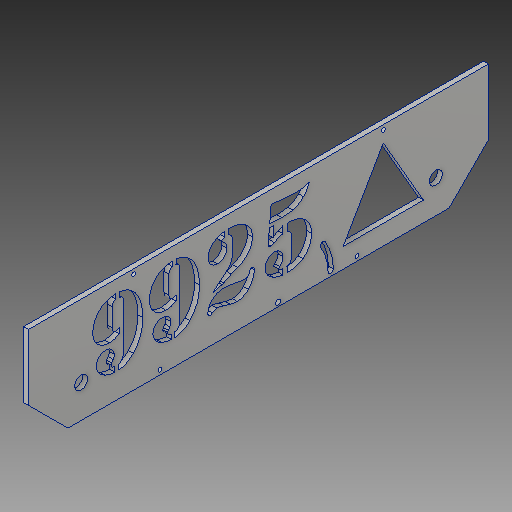
# Autodesk Inventor part: DriveTrain3.0
Saved by Autodesk Inventor 2019 (Build 230136000, 136)
## iProperties
Created: 2017-07-22
Part Number: DriveTrain3.0
Material: Aluminum 6061
Document SubType Name: Modeling
Designer: User
Density: 2.7 g/cm^3
Appearance: Aluminum - Flat
Mass: 590.045 g
Surface Area: 982.684 cm^2
Volume: 218.535 cm^3
Author: User
Autodesk Inventor part; units mm, degrees
ref_plane "YZ Plane" through (0, 0, 0) normal (1, 0, 0) x (0, 1, 0)
ref_plane "XZ Plane" through (0, 0, 0) normal (0, 1, 0) x (-1, 0, 0)
ref_plane "XY Plane" through (0, 0, 0) normal (0, 0, 1) x (1, 0, 0)
sketch "Sketch1" plane through (0, 0, 0) normal (1, 0, 0) x (0, 1, 0)
  line L0 (0, 0) -> (101.6, 0)
  line L1 (101.6, 0) -> (101.6, -444.5)
  line L2 (101.6, -444.5) -> (0, -444.5)
  line L3 (0, -444.5) -> (0, 0)
  circle A0 centre (31.75, -50.8) radius 6.3627
  circle A1 centre (31.75, -393.7) radius 6.3627
  circle A2 centre (86.2838, -165.5318) radius 1.5875
  circle A3 centre (70.2818, -165.5318) radius 1.5875
  circle A4 centre (15.3162, -278.9682) radius 1.5875
  circle A5 centre (31.3182, -278.9682) radius 1.5875
  dimension "d0" = 101.6
  dimension "d1" = 444.5
  dimension "d2" = 12.7254
  dimension "d3" = 31.75
  dimension "d4" = 50.8
  dimension "d5" = 50.8
  dimension "d22" = 165.5318
  dimension "d23" = 3.175
  dimension "d24" = 15.3162
  dimension "d25" = 3.175
  dimension "d26" = 16.002
  dimension "d27" = 165.5318
  dimension "d28" = 3.175
  dimension "d29" = 15.3162
  dimension "d30" = 165.5318
  dimension "d31" = 3.175
  dimension "d32" = 16.002
  dimension "d33" = 165.5318
  constraints: 8 end point, 6 centre point, 2 parallel, 1 horizontal, 1 perpendicular
  measures "d0" distance of L1.end L2.end
  measures "d1" distance of L0.end L1.end
  measures "d2" diameter of A0
  measures "d3" distance from line of L3 A0.centre
  measures "d4" distance from line of L0 A0.centre
  measures "d5" distance from line of L2 A1.centre
  measures "d22" distance from line of L0 A2.centre
  measures "d23" diameter of A2
  measures "d24" distance from line of L1 A2.centre
  measures "d25" diameter of A3
  measures "d26" distance of A2.centre A3.centre
  measures "d27" distance from line of L0 A3.centre
  measures "d28" diameter of A4
  measures "d29" distance from line of L3 A4.centre
  measures "d30" distance from line of L2 A4.centre
  measures "d31" diameter of A5
  measures "d32" distance of A5.centre A4.centre
  measures "d33" distance from line of L2 A5.centre
extrude "Extrusion1" add sketch "Sketch1" along normal blind 4.7625 contours L0 L1 L2 L3 | A2 | A3 | A4 | A5
chamfer "Chamfer1" distance 38.1 angle 45 1 edges at (2.3813, 0, 0)
chamfer "Chamfer2" distance 38.1 angle 45 1 edges at (2.3813, 0, -444.5)
sketch "Sketch8" plane through (4.7625, 0, 0) normal (1, 0, 0) x (0, 0, -1)
  line L0 (444.5, 38.1) -> (406.4, 0) projected
  line L1 (444.5, 38.1) -> (444.5, 101.6) projected
  line L2 (444.5, 101.6) -> (0, 101.6) projected
  line L3 (0, 101.6) -> (0, 38.1) projected
  line L4 (38.1, 0) -> (0, 38.1) projected
  line L5 (38.1, 0) -> (406.4, 0) projected
  circle A0 centre (393.7, 31.75) radius 6.3627 projected
  circle A1 centre (50.8, 31.75) radius 6.3627 projected
  point P0 (0, 0)
  point P1 (101.6, 97.155)
  point P2 (342.9, 97.155)
  point P3 (127, 4.445)
  point P4 (317.5, 4.445)
  dimension "d110" = 4.445
  dimension "d111" = 4.445
  dimension "d112" = 101.6
  dimension "d113" = 101.6
  dimension "d114" = 4.445
  dimension "d115" = 4.445
  dimension "d123" = 127
  dimension "d124" = 127
  measures "d110" distance from line of L2 point (342.9, 97.155)
  measures "d111" distance from line of L2 point (101.6, 97.155)
  measures "d112" distance from line of L3 point (101.6, 97.155)
  measures "d113" distance from line of L1 point (342.9, 97.155)
  measures "d114" distance from line of L5 point (317.5, 4.445)
  measures "d115" distance from line of L5 point (127, 4.445)
  measures "d123" distance from line of L1 point (317.5, 4.445)
  measures "d124" distance from line of L3 point (127, 4.445)
hole "Hole3" at (4.7625, 97.155, -101.6) at (4.7625, 97.155, -342.9) at (4.7625, 4.445, -127) at (4.7625, 4.445, -317.5) direction (-1, 0, 0) diameter 3.81 depth 25.4 tip angle 118
sketch "Sketch9" plane through (4.7625, 0, 0) normal (1, 0, 0) x (0, 0, -1)
  line L0 (444.5, 38.1) -> (444.5, 101.6) projected
  line L1 (38.1, 0) -> (406.4, 0) projected
  arc A0 (292.0841, 5.08) -> (284.536, 30.48) centre (241.3, 3.81) ccw construction
  arc A1 (294.6233, 5.1435) -> (286.6978, 31.8135) centre (241.3, 3.81) ccw
  arc A2 (289.5449, 5.0165) -> (282.3742, 29.1465) centre (241.3, 3.81) ccw
  arc A3 (289.5449, 5.0165) -> (294.6233, 5.1435) centre (292.0841, 5.08) ccw
  arc A4 (286.6978, 31.8135) -> (282.3742, 29.1465) centre (284.536, 30.48) ccw
  point P0 (0, 0)
  dimension "d125" = 203.2
  dimension "d126" = 3.81
  dimension "d134" = 50.8
  dimension "d135" = 5.08
  dimension "d139" = 5.08
  dimension "d140" = 25.4
  constraints: 10 point on circle, 5 centre point, 4 tangent, 1 coincident
  measures "d125" distance from line of L0 point (241.3, 3.81)
  measures "d126" distance from line of point (241.3, 3.81) L1
  measures "d134" radius of A0
  measures "d135" diameter of A4
  measures "d139" distance from line of L1 A0.start
  measures "d140" vertical distance of A0.start A0.end
hole "Hole4" at (4.7625, 3.81, -241.3) direction (-1, 0, 0) diameter 5.08 end through all
extrude "Extrusion6" cut sketch "Sketch9" against normal through all
sketch "Sketch10" plane through (4.7625, 0, 0) normal (1, 0, 0) x (0, 0, -1)
  line L0 (59.5129, 89.2474) -> (313.2288, 89.2474) construction
  line L1 (313.2288, 89.2474) -> (313.2288, 0) construction
  line L2 (313.2288, 0) -> (59.5129, 0) construction
  line L3 (59.5129, 0) -> (59.5129, 89.2474) construction
  line L4 (86.7981, 24.204) -> (86.7981, 28.8893)
  spline S0 degree 2 poles (86.7981, 28.8893) (88.2863, 29.3303) (89.8297, 30.3776) (90.381, 31.3698) knots 0 0 0 1 2 2 2
  spline S1 degree 2 poles (90.381, 31.3698) (91.5385, 33.299) (91.5385, 35.6141) knots 0 0 0 1 1 1
  line L5 (91.5385, 35.6141) -> (91.5385, 78.5538)
  spline S2 degree 2 poles (91.5385, 78.5538) (91.5385, 80.7036) (91.2629, 82.5226) (90.7668, 83.184) knots 0 0 0 1 2 2 2
  spline S3 degree 2 poles (90.7668, 83.184) (89.9951, 84.1211) (87.9005, 84.7274) knots 0 0 0 1 1 1
  line L6 (87.9005, 84.7274) -> (87.9005, 89.2474)
  spline S4 degree 2 poles (87.9005, 89.2474) (92.3653, 88.8064) (100.1926, 84.4518) (103.2243, 80.7587) knots 0 0 0 1 2 2 2
  spline S5 degree 2 poles (103.2243, 80.7587) (106.6969, 76.6797) (110.4452, 63.8364) (110.4452, 56.3398) knots 0 0 0 1 2 2 2
  spline S6 degree 2 poles (110.4452, 56.3398) (110.4452, 40.3546) (101.295, 31.0391) knots 0 0 0 1 1 1
  spline S7 degree 2 poles (101.295, 31.0391) (98.0429, 27.7869) (90.4912, 24.204) (86.7981, 24.204) knots 0 0 0 1 2 2 2
  line L7 (87.9005, 59.3715) -> (87.9005, 54.0247)
  spline S8 degree 2 poles (87.9005, 54.0247) (82.8293, 51.2687) (78.0889, 51.2687) knots 0 0 0 1 1 1
  spline S9 degree 2 poles (78.0889, 51.2687) (75.1674, 51.2687) (69.3797, 53.5286) (67.1748, 55.4579) knots 0 0 0 1 2 2 2
  spline S10 degree 2 poles (67.1748, 55.4579) (64.7495, 57.6628) (62.0485, 64.0569) (62.0485, 67.6949) knots 0 0 0 1 2 2 2
  spline S11 degree 2 poles (62.0485, 67.6949) (62.0485, 72.8763) (66.8441, 82.5777) (70.8128, 85.3338) knots 0 0 0 1 2 2 2
  spline S12 degree 2 poles (70.8128, 85.3338) (76.5455, 89.2474) (84.3727, 89.2474) knots 0 0 0 1 1 1
  line L8 (84.3727, 89.2474) -> (84.3727, 84.7274)
  spline S13 degree 2 poles (84.3727, 84.7274) (82.5537, 84.2313) (80.9552, 82.1918) (80.9552, 80.2075) knots 0 0 0 1 2 2 2
  line L9 (80.9552, 80.2075) -> (80.9552, 62.5134)
  spline S14 degree 2 poles (80.9552, 62.5134) (80.9552, 60.4188) (82.7191, 58.0486) (84.2073, 58.1037) knots 0 0 0 1 2 2 2
  spline S15 degree 2 poles (84.2073, 58.1037) (85.6405, 58.1588) (87.9005, 59.3715) knots 0 0 0 1 1 1
  line L10 (83.3254, 28.8893) -> (83.3254, 24.204)
  spline S16 degree 2 poles (83.3254, 24.204) (78.6952, 24.204) (73.9547, 26.4088) knots 0 0 0 1 1 1
  spline S17 degree 2 poles (73.9547, 26.4088) (69.986, 28.3381) (65.466, 34.4015) (65.466, 37.9292) knots 0 0 0 1 2 2 2
  spline S18 degree 2 poles (65.466, 37.9292) (65.466, 41.7878) (70.6475, 47.0243) (74.5611, 47.0243) knots 0 0 0 1 2 2 2
  spline S19 degree 2 poles (74.5611, 47.0243) (78.0337, 47.0243) (82.8844, 42.5043) (82.8844, 39.3073) knots 0 0 0 1 2 2 2
  spline S20 degree 2 poles (82.8844, 39.3073) (82.8844, 37.1024) (81.8371, 35.559) knots 0 0 0 1 1 1
  line L11 (81.8371, 35.559) -> (80.3488, 33.4644)
  spline S21 degree 2 poles (80.3488, 33.4644) (79.7425, 32.5825) (79.7425, 31.8108) knots 0 0 0 1 1 1
  spline S22 degree 2 poles (79.7425, 31.8108) (79.7425, 30.4878) (81.1757, 29.4957) knots 0 0 0 1 1 1
  spline S23 degree 2 poles (81.1757, 29.4957) (81.8922, 28.9996) (83.3254, 28.8893) knots 0 0 0 1 1 1
  line L12 (141.5337, 24.204) -> (141.5337, 28.8893)
  spline S24 degree 2 poles (141.5337, 28.8893) (143.022, 29.3303) (144.5654, 30.3776) (145.1166, 31.3698) knots 0 0 0 1 2 2 2
  spline S25 degree 2 poles (145.1166, 31.3698) (146.2742, 33.299) (146.2742, 35.6141) knots 0 0 0 1 1 1
  line L13 (146.2742, 35.6141) -> (146.2742, 78.5538)
  spline S26 degree 2 poles (146.2742, 78.5538) (146.2742, 80.7036) (145.9986, 82.5226) (145.5025, 83.184) knots 0 0 0 1 2 2 2
  spline S27 degree 2 poles (145.5025, 83.184) (144.7308, 84.1211) (142.6362, 84.7274) knots 0 0 0 1 1 1
  line L14 (142.6362, 84.7274) -> (142.6362, 89.2474)
  spline S28 degree 2 poles (142.6362, 89.2474) (147.101, 88.8064) (154.9283, 84.4518) (157.96, 80.7587) knots 0 0 0 1 2 2 2
  spline S29 degree 2 poles (157.96, 80.7587) (161.4326, 76.6797) (165.1809, 63.8364) (165.1809, 56.3398) knots 0 0 0 1 2 2 2
  spline S30 degree 2 poles (165.1809, 56.3398) (165.1809, 40.3546) (156.0307, 31.0391) knots 0 0 0 1 1 1
  spline S31 degree 2 poles (156.0307, 31.0391) (152.7785, 27.7869) (145.2269, 24.204) (141.5337, 24.204) knots 0 0 0 1 2 2 2
  line L15 (142.6362, 59.3715) -> (142.6362, 54.0247)
  spline S32 degree 2 poles (142.6362, 54.0247) (137.565, 51.2687) (132.8245, 51.2687) knots 0 0 0 1 1 1
  spline S33 degree 2 poles (132.8245, 51.2687) (129.9031, 51.2687) (124.1153, 53.5286) (121.9105, 55.4579) knots 0 0 0 1 2 2 2
  spline S34 degree 2 poles (121.9105, 55.4579) (119.4851, 57.6628) (116.7842, 64.0569) (116.7842, 67.6949) knots 0 0 0 1 2 2 2
  spline S35 degree 2 poles (116.7842, 67.6949) (116.7842, 72.8763) (121.5797, 82.5777) (125.5485, 85.3338) knots 0 0 0 1 2 2 2
  spline S36 degree 2 poles (125.5485, 85.3338) (131.2811, 89.2474) (139.1084, 89.2474) knots 0 0 0 1 1 1
  line L16 (139.1084, 89.2474) -> (139.1084, 84.7274)
  spline S37 degree 2 poles (139.1084, 84.7274) (137.2894, 84.2313) (135.6909, 82.1918) (135.6909, 80.2075) knots 0 0 0 1 2 2 2
  line L17 (135.6909, 80.2075) -> (135.6909, 62.5134)
  spline S38 degree 2 poles (135.6909, 62.5134) (135.6909, 60.4188) (137.4547, 58.0486) (138.943, 58.1037) knots 0 0 0 1 2 2 2
  spline S39 degree 2 poles (138.943, 58.1037) (140.3762, 58.1588) (142.6362, 59.3715) knots 0 0 0 1 1 1
  line L18 (138.0611, 28.8893) -> (138.0611, 24.204)
  spline S40 degree 2 poles (138.0611, 24.204) (133.4309, 24.204) (128.6904, 26.4088) knots 0 0 0 1 1 1
  spline S41 degree 2 poles (128.6904, 26.4088) (124.7217, 28.3381) (120.2017, 34.4015) (120.2017, 37.9292) knots 0 0 0 1 2 2 2
  spline S42 degree 2 poles (120.2017, 37.9292) (120.2017, 41.7878) (125.3831, 47.0243) (129.2968, 47.0243) knots 0 0 0 1 2 2 2
  spline S43 degree 2 poles (129.2968, 47.0243) (132.7694, 47.0243) (137.6201, 42.5043) (137.6201, 39.3073) knots 0 0 0 1 2 2 2
  spline S44 degree 2 poles (137.6201, 39.3073) (137.6201, 37.1024) (136.5728, 35.559) knots 0 0 0 1 1 1
  line L19 (136.5728, 35.559) -> (135.0845, 33.4644)
  spline S45 degree 2 poles (135.0845, 33.4644) (134.4782, 32.5825) (134.4782, 31.8108) knots 0 0 0 1 1 1
  spline S46 degree 2 poles (134.4782, 31.8108) (134.4782, 30.4878) (135.9113, 29.4957) knots 0 0 0 1 1 1
  spline S47 degree 2 poles (135.9113, 29.4957) (136.6279, 28.9996) (138.0611, 28.8893) knots 0 0 0 1 1 1
  line L20 (193.5685, 84.1762) -> (193.5685, 89.2474)
  line L21 (193.5685, 89.2474) -> (194.8363, 89.2474)
  spline S48 degree 2 poles (194.8363, 89.2474) (199.6869, 89.2474) (208.4513, 86.0503) (211.3727, 83.184) knots 0 0 0 1 2 2 2
  spline S49 degree 2 poles (211.3727, 83.184) (216.3336, 78.3884) (216.3336, 71.1124) knots 0 0 0 1 1 1
  spline S50 degree 2 poles (216.3336, 71.1124) (216.3336, 64.8286) (208.9474, 55.1272) (202.1123, 52.3711) knots 0 0 0 1 2 2 2
  line L22 (202.1123, 52.3711) -> (196.0489, 49.9457)
  spline S51 degree 2 poles (196.0489, 49.9457) (193.4031, 48.8984) (188.5524, 46.2526) knots 0 0 0 1 1 1
  line L23 (188.5524, 46.2526) -> (187.1744, 45.4258)
  spline S52 degree 2 poles (187.1744, 45.4258) (185.3002, 45.4258) (181.8276, 44.4336) (178.5754, 43.0555) knots 0 0 0 1 2 2 2
  spline S53 degree 2 poles (178.5754, 43.0555) (180.2842, 45.3155) (183.6466, 48.5677) (187.0641, 51.2135) knots 0 0 0 1 2 2 2
  spline S54 degree 2 poles (187.0641, 51.2135) (191.4187, 54.5759) (194.4504, 57.6076) (195.5528, 59.6471) knots 0 0 0 1 2 2 2
  spline S55 degree 2 poles (195.5528, 59.6471) (196.6001, 61.6866) (197.5923, 67.1988) (197.5923, 71.4431) knots 0 0 0 1 2 2 2
  spline S56 degree 2 poles (197.5923, 71.4431) (197.5923, 78.8845) (196.2694, 81.4753) knots 0 0 0 1 1 1
  spline S57 degree 2 poles (196.2694, 81.4753) (195.7733, 82.5226) (194.6158, 83.625) (193.5685, 84.1762) knots 0 0 0 1 2 2 2
  spline S58 degree 2 poles (215.8927, 45.6463) (216.94, 45.7014) (218.2629, 43.9375) (218.2629, 42.5043) knots 0 0 0 1 2 2 2
  spline S59 degree 2 poles (218.2629, 42.5043) (218.2629, 39.2522) (214.8454, 31.3147) (212.4751, 28.8893) knots 0 0 0 1 2 2 2
  spline S60 degree 2 poles (212.4751, 28.8893) (210.4356, 26.7947) (204.4274, 24.204) (201.7264, 24.204) knots 0 0 0 1 2 2 2
  spline S61 degree 2 poles (201.7264, 24.204) (198.4743, 24.204) (194.8363, 25.2513) knots 0 0 0 1 1 1
  line L24 (194.8363, 25.2513) -> (188.7178, 27.0703)
  spline S62 degree 2 poles (188.7178, 27.0703) (183.5363, 28.5586) (181.9929, 28.5586) knots 0 0 0 1 1 1
  spline S63 degree 2 poles (181.9929, 28.5586) (179.9534, 28.5586) (177.6935, 26.6293) knots 0 0 0 1 1 1
  spline S64 degree 2 poles (177.6935, 26.6293) (176.2603, 25.4167) (175.4886, 25.4167) knots 0 0 0 1 1 1
  spline S65 degree 2 poles (175.4886, 25.4167) (174.4413, 25.4167) (173.2837, 26.7947) (173.2837, 28.1176) knots 0 0 0 1 2 2 2
  spline S66 degree 2 poles (173.2837, 28.1176) (173.2837, 30.5981) (175.5988, 35.8346) (177.5832, 37.7639) knots 0 0 0 1 2 2 2
  spline S67 degree 2 poles (177.5832, 37.7639) (181.8276, 41.898) (189.1036, 41.898) knots 0 0 0 1 1 1
  spline S68 degree 2 poles (189.1036, 41.898) (192.5211, 41.898) (198.3089, 40.8507) knots 0 0 0 1 1 1
  spline S69 degree 2 poles (198.3089, 40.8507) (206.6874, 39.2522) (209.223, 39.2522) knots 0 0 0 1 1 1
  spline S70 degree 2 poles (209.223, 39.2522) (211.483, 39.2522) (212.5303, 40.3546) knots 0 0 0 1 1 1
  spline S71 degree 2 poles (212.5303, 40.3546) (212.9161, 40.7956) (213.3571, 41.8429) (213.6878, 43.276) knots 0 0 0 1 2 2 2
  spline S72 degree 2 poles (213.6878, 43.276) (214.1839, 45.536) (215.8927, 45.6463) knots 0 0 0 1 1 1
  line L25 (189.4343, 89.1371) -> (189.4343, 84.1762)
  spline S73 degree 2 poles (189.4343, 84.1762) (188.1114, 83.9006) (186.4578, 82.9084) (186.5129, 82.3572) knots 0 0 0 1 2 2 2
  spline S74 degree 2 poles (186.5129, 82.3572) (186.6231, 81.7509) (187.7807, 80.9792) knots 0 0 0 1 1 1
  spline S75 degree 2 poles (187.7807, 80.9792) (189.8753, 79.546) (191.7494, 76.1836) (191.7494, 73.8134) knots 0 0 0 1 2 2 2
  spline S76 degree 2 poles (191.7494, 73.8134) (191.7494, 70.2856) (186.4027, 65.1593) (182.7646, 65.1593) knots 0 0 0 1 2 2 2
  spline S77 degree 2 poles (182.7646, 65.1593) (178.7959, 65.1593) (173.5042, 70.6163) (173.5042, 74.6402) knots 0 0 0 1 2 2 2
  spline S78 degree 2 poles (173.5042, 74.6402) (173.5042, 78.4436) (178.1344, 85.0582) (182.0481, 86.9874) knots 0 0 0 1 2 2 2
  spline S79 degree 2 poles (182.0481, 86.9874) (184.5836, 88.2001) (189.4343, 89.1371) knots 0 0 0 1 1 1
  line L26 (249.8475, 58.8754) -> (249.8475, 65.6003)
  spline S80 degree 2 poles (249.8475, 65.6003) (254.6431, 65.6003) (261.1475, 64.112) (264.124, 62.3481) knots 0 0 0 1 2 2 2
  spline S81 degree 2 poles (264.124, 62.3481) (273.4947, 56.8911) (273.4947, 45.3707) knots 0 0 0 1 1 1
  spline S82 degree 2 poles (273.4947, 45.3707) (273.4947, 39.8034) (269.1952, 30.9839) (265.2816, 28.2279) knots 0 0 0 1 2 2 2
  spline S83 degree 2 poles (265.2816, 28.2279) (262.4704, 26.4088) (255.0841, 24.204) (251.4461, 24.204) knots 0 0 0 1 2 2 2
  line L27 (251.4461, 24.204) -> (249.9578, 24.204)
  line L28 (249.9578, 24.204) -> (249.9578, 29.4405)
  spline S84 degree 2 poles (249.9578, 29.4405) (251.4461, 29.8815) (253.1548, 31.3698) (253.706, 32.6376) knots 0 0 0 1 2 2 2
  spline S85 degree 2 poles (253.706, 32.6376) (254.0919, 33.4093) (254.588, 36.7166) (254.588, 38.26) knots 0 0 0 1 2 2 2
  line L29 (254.588, 38.26) -> (254.588, 50.1662)
  spline S86 degree 2 poles (254.588, 50.1662) (254.588, 54.2452) (252.6587, 57.8281) (249.8475, 58.8754) knots 0 0 0 1 2 2 2
  line L30 (233.1457, 73.8685) -> (234.4686, 89.2474)
  spline S87 degree 2 poles (234.4686, 89.2474) (236.012, 89.082) (236.2876, 89.0269) knots 0 0 0 1 1 1
  line L31 (236.2876, 89.0269) -> (245.6583, 87.8142)
  spline S88 degree 2 poles (245.6583, 87.8142) (250.6744, 87.0976) (257.5646, 87.0976) knots 0 0 0 1 1 1
  spline S89 degree 2 poles (257.5646, 87.0976) (262.2499, 87.0976) (267.9825, 88.0347) (271.1796, 89.2474) knots 0 0 0 1 2 2 2
  spline S90 degree 2 poles (271.1796, 89.2474) (270.1874, 86.0503) (267.8723, 81.9713) (265.7777, 79.8767) knots 0 0 0 1 2 2 2
  spline S91 degree 2 poles (265.7777, 79.8767) (263.5177, 77.6167) (258.1158, 74.4748) (255.4148, 73.8685) knots 0 0 0 1 2 2 2
  spline S92 degree 2 poles (255.4148, 73.8685) (251.2807, 72.9314) (244.7764, 72.9314) knots 0 0 0 1 1 1
  spline S93 degree 2 poles (244.7764, 72.9314) (238.8784, 72.9314) (233.1457, 73.8685) knots 0 0 0 1 1 1
  line L32 (245.9339, 29.4405) -> (245.9339, 24.3142)
  spline S94 degree 2 poles (245.9339, 24.3142) (241.0281, 24.645) (236.8389, 26.8498) knots 0 0 0 1 1 1
  spline S95 degree 2 poles (236.8389, 26.8498) (232.9252, 28.8893) (228.6809, 34.7873) (228.6809, 38.3151) knots 0 0 0 1 2 2 2
  spline S96 degree 2 poles (228.6809, 38.3151) (228.6809, 42.339) (233.8623, 47.7409) (237.7759, 47.7409) knots 0 0 0 1 2 2 2
  spline S97 degree 2 poles (237.7759, 47.7409) (241.0832, 47.7409) (245.989, 42.8902) (245.989, 39.5829) knots 0 0 0 1 2 2 2
  spline S98 degree 2 poles (245.989, 39.5829) (245.989, 37.7088) (244.1149, 33.8503) (242.792, 32.8581) knots 0 0 0 1 2 2 2
  spline S99 degree 2 poles (242.792, 32.8581) (241.6896, 32.0312) (241.6896, 31.5352) knots 0 0 0 1 1 1
  spline S100 degree 2 poles (241.6896, 31.5352) (241.6896, 30.7634) (243.9495, 29.661) (245.9339, 29.4405) knots 0 0 0 1 2 2 2
  line L33 (232.815, 70.2856) -> (237.1145, 69.8446)
  line L34 (237.1145, 69.8446) -> (236.2876, 60.1983)
  spline S101 degree 2 poles (236.2876, 60.1983) (239.0437, 62.4583) (243.3432, 64.7734) (245.9339, 65.4349) knots 0 0 0 1 2 2 2
  line L35 (245.9339, 65.4349) -> (245.9339, 58.8754)
  spline S102 degree 2 poles (245.9339, 58.8754) (240.973, 57.7179) (237.5554, 55.6233) knots 0 0 0 1 1 1
  spline S103 degree 2 poles (237.5554, 55.6233) (235.3506, 54.2452) (234.3033, 54.2452) knots 0 0 0 1 1 1
  spline S104 degree 2 poles (234.3033, 54.2452) (233.0355, 54.2452) (231.6023, 55.6233) (231.6023, 56.7808) knots 0 0 0 1 2 2 2
  spline S105 degree 2 poles (231.6023, 56.7808) (231.6023, 57.332) (231.6574, 58.0486) knots 0 0 0 1 1 1
  line L36 (231.6574, 58.0486) -> (232.815, 70.2856)
  point P0 (0, 0)
  constraints: 2 other
extrude "Extrusion7" cut sketch "Sketch10" against normal through all
sketch "Sketch11" plane through (4.7625, 0, 0) normal (1, 0, 0) x (0, 0, -1)
  line L0 (342.9, 86.2756) -> (381.7127, 19.05)
  line L1 (381.7127, 19.05) -> (304.0873, 19.05)
  line L2 (304.0873, 19.05) -> (342.9, 86.2756)
  line L3 (38.1, 0) -> (406.4, 0) projected
  line L4 (444.5, 101.6) -> (0, 101.6) projected
  line L5 (444.5, 38.1) -> (444.5, 101.6) projected
  point P0 (0, 0)
  point P1 (342.9, 41.4585)
  dimension "d143" = 19.05
  dimension "d144" = 19.05
  dimension "d145" = 15.3244
  dimension "d146" = 101.6
  constraints: 6 end point, 7 other
  measures "d143" distance from line of L3 L0.end
  measures "d144" distance from line of L3 L1.end
  measures "d145" distance from line of L4 L0.start
  measures "d146" distance from line of L5 L0.start
extrude "Extrusion8" cut sketch "Sketch11" against normal through all
sketch "Sketch12" plane through (4.7625, 0, 0) normal (1, 0, 0) x (0, 0, -1)
  circle A0 centre (331.5884, 34.94) radius 5.08
  line L0 (330.888, 39.9715) -> (332.158, 41.102)
  line L1 (332.158, 41.102) -> (333.428, 39.6753)
  line L2 (328.4661, 38.9472) -> (329.0007, 40.5612)
  line L3 (329.0007, 40.5612) -> (330.8139, 39.9606)
  line L4 (326.8808, 36.8492) -> (326.5368, 38.5143)
  line L5 (326.5368, 38.5143) -> (328.4074, 38.9007)
  line L6 (326.557, 34.2396) -> (325.4265, 35.5096)
  line L7 (325.4265, 35.5096) -> (326.8532, 36.7796)
  line L8 (327.5813, 31.8177) -> (325.9672, 32.3523)
  line L9 (325.9672, 32.3523) -> (326.5678, 34.1655)
  line L10 (329.6793, 30.2324) -> (328.0142, 29.8884)
  line L11 (328.0142, 29.8884) -> (327.6277, 31.759)
  line L12 (332.2889, 29.9085) -> (331.0189, 28.7781)
  line L13 (331.0189, 28.7781) -> (329.7489, 30.2048)
  line L14 (334.7108, 30.9329) -> (334.1762, 29.3188)
  line L15 (334.1762, 29.3188) -> (332.363, 29.9194)
  line L16 (336.296, 33.0309) -> (336.6401, 31.3658)
  line L17 (336.6401, 31.3658) -> (334.7695, 30.9793)
  line L18 (336.6199, 35.6405) -> (337.7504, 34.3705)
  line L19 (337.7504, 34.3705) -> (336.3237, 33.1005)
  line L20 (335.5956, 38.0624) -> (337.2096, 37.5278)
  line L21 (337.2096, 37.5278) -> (336.609, 35.7145)
  line L22 (333.4976, 39.6476) -> (335.1627, 39.9917)
  line L23 (335.1627, 39.9917) -> (335.5492, 38.1211)
  line L24 (304.0873, 19.05) -> (342.9, 86.2756) projected
  line L25 (342.9, 86.2756) -> (381.7127, 19.05) projected
  circle A1 centre (342.9, 58.6942) radius 5.08
  line L26 (342.1996, 63.7257) -> (343.4696, 64.8562)
  line L27 (343.4696, 64.8562) -> (344.7396, 63.4295)
  line L28 (339.7777, 62.7014) -> (340.3123, 64.3154)
  line L29 (340.3123, 64.3154) -> (342.1255, 63.7149)
  line L30 (338.1924, 60.6034) -> (337.8484, 62.2685)
  line L31 (337.8484, 62.2685) -> (339.7189, 62.655)
  line L32 (337.8685, 57.9938) -> (336.738, 59.2638)
  line L33 (336.738, 59.2638) -> (338.1648, 60.5338)
  line L34 (338.8928, 55.5719) -> (337.2788, 56.1065)
  line L35 (337.2788, 56.1065) -> (337.8794, 57.9197)
  line L36 (340.9909, 53.9866) -> (339.3258, 53.6426)
  line L37 (339.3258, 53.6426) -> (338.9393, 55.5132)
  line L38 (343.6004, 53.6628) -> (342.3304, 52.5323)
  line L39 (342.3304, 52.5323) -> (341.0604, 53.959)
  line L40 (346.0223, 54.6871) -> (345.4877, 53.073)
  line L41 (345.4877, 53.073) -> (343.6745, 53.6736)
  line L42 (347.6076, 56.7851) -> (347.9516, 55.12)
  line L43 (347.9516, 55.12) -> (346.0811, 54.7335)
  line L44 (347.9315, 59.3947) -> (349.062, 58.1247)
  line L45 (349.062, 58.1247) -> (347.6352, 56.8547)
  line L46 (346.9072, 61.8166) -> (348.5212, 61.282)
  line L47 (348.5212, 61.282) -> (347.9206, 59.4688)
  line L48 (344.8091, 63.4019) -> (346.4742, 63.7459)
  line L49 (346.4742, 63.7459) -> (346.8607, 61.8753)
  circle A2 centre (359.7518, 34.2396) radius 5.08
  line L50 (359.0513, 39.2711) -> (360.3213, 40.4015)
  line L51 (360.3213, 40.4015) -> (361.5913, 38.9748)
  line L52 (356.6294, 38.2467) -> (357.1641, 39.8608)
  line L53 (357.1641, 39.8608) -> (358.9773, 39.2602)
  line L54 (355.0442, 36.1487) -> (354.7001, 37.8138)
  line L55 (354.7001, 37.8138) -> (356.5707, 38.2003)
  line L56 (354.7203, 33.5391) -> (353.5898, 34.8091)
  line L57 (353.5898, 34.8091) -> (355.0166, 36.0791)
  line L58 (355.7446, 31.1172) -> (354.1306, 31.6518)
  line L59 (354.1306, 31.6518) -> (354.7312, 33.4651)
  line L60 (357.8427, 29.532) -> (356.1776, 29.1879)
  line L61 (356.1776, 29.1879) -> (355.7911, 31.0585)
  line L62 (360.4522, 29.2081) -> (359.1822, 28.0776)
  line L63 (359.1822, 28.0776) -> (357.9122, 29.5043)
  line L64 (362.8741, 30.2324) -> (362.3395, 28.6184)
  line L65 (362.3395, 28.6184) -> (360.5263, 29.219)
  line L66 (364.4594, 32.3304) -> (364.8034, 30.6653)
  line L67 (364.8034, 30.6653) -> (362.9328, 30.2789)
  line L68 (364.7833, 34.94) -> (365.9138, 33.67)
  line L69 (365.9138, 33.67) -> (364.487, 32.4)
  line L70 (363.759, 37.3619) -> (365.373, 36.8273)
  line L71 (365.373, 36.8273) -> (364.7724, 35.0141)
  line L72 (361.6609, 38.9472) -> (363.326, 39.2912)
  line L73 (363.326, 39.2912) -> (363.7125, 37.4206)
  line L74 (339.7189, 62.655) -> (334.9264, 72.465)
  line L75 (338.1924, 60.6034) -> (333.4837, 69.9661)
  line L76 (346.9072, 61.8166) -> (350.6482, 72.8553)
  line L77 (347.9315, 59.3947) -> (351.8054, 70.851)
  line L78 (363.759, 37.3619) -> (369.295, 40.5581)
  line L79 (364.7833, 34.94) -> (376.1199, 28.737)
  line L80 (360.4522, 29.2081) -> (360.4522, 19.05)
  line L81 (381.7127, 19.05) -> (304.0873, 19.05) projected
  line L82 (357.9122, 29.5043) -> (354.8448, 19.05)
  line L83 (329.7489, 30.2048) -> (311.4116, 19.05)
  line L84 (332.2889, 29.9085) -> (316.7866, 19.05)
  line L85 (328.4074, 38.9007) -> (310.9176, 30.8805)
  line L86 (326.8532, 36.7796) -> (309.4951, 28.4166)
  point P0 (0, 0)
  dimension "d149" = 10.16
  dimension "d152" = 1.27
  dimension "d153" = 1.27
  dimension "d154" = 6.162
  dimension "d157" = 360
  dimension "d161" = 10.16
  dimension "d162" = 1.27
  dimension "d163" = 1.27
  dimension "d164" = 6.162
  dimension "d165" = 360
  dimension "d168" = 10.16
  dimension "d169" = 1.27
  dimension "d170" = 1.27
  dimension "d171" = 6.162
  dimension "d172" = 360
  constraints: 168 end point, 12 point on line, 6 point on circle, 4 perpendicular, 3 centre point, 1 coincident, 1 vertical, 183 other
  measures "d149" diameter of A0
  measures "d152" horizontal distance of L0.end L1.end
  measures "d153" horizontal distance of L0.start L0.end
  measures "d154" vertical distance of A0.centre L0.end
  measures "d161" diameter of A1
  measures "d162" horizontal distance of L26.end L27.end
  measures "d163" horizontal distance of L26.start L26.end
  measures "d164" vertical distance of A1.centre L26.end
  measures "d168" diameter of A2
  measures "d169" horizontal distance of L50.end L51.end
  measures "d170" horizontal distance of L50.start L50.end
  measures "d171" vertical distance of A2.centre L50.end
equation "\"d110\" = d111"
equation "\"d112\" = d113"
equation "\"d114\" = d111"
equation "\"d115\" = d111"
equation "\"d124\" = d123"
equation "\"d144\" = d143"
equation "\"d153\" = d152"
equation "\"d163\" = d162"
equation "\"d170\" = d169"
body "Solid1"
